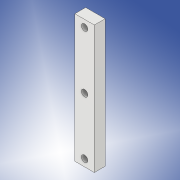
# Autodesk Inventor part: SJ017
Saved by Autodesk Inventor 2017 SP1 (Build 210196100, 196)
## iProperties
Created: 2017-07-22
Part Number: SJ017
Material: ABS Plastic
Document SubType Name: Modeling
Designer: Zach
Density: 1.06 g/cm^3
Appearance: CR White
Author: Zach
Autodesk Inventor part; units mm, degrees
ref_plane "YZ Plane" through (0, 0, 0) normal (1, 0, 0) x (0, 1, 0)
ref_plane "XZ Plane" through (0, 0, 0) normal (0, 1, 0) x (-1, 0, 0)
ref_plane "XY Plane" through (0, 0, 0) normal (0, 0, 1) x (1, 0, 0)
sketch "Sketch1" plane through (0, 0, 0) normal (0, 0, 1) x (1, 0, 0)
  line L0 (0, 0) -> (9, 0)
  line L1 (9, 0) -> (9, 59)
  line L2 (9, 59) -> (0, 59)
  line L3 (0, 59) -> (0, 0)
  circle A0 centre (4.5, 55.75) radius 1.5
  circle A1 centre (4.5, 3.25) radius 1.5
  line L4 (4.5, 55.75) -> (4.5, 3.25) construction
  circle A2 centre (4.5, 29.5) radius 1.5
  point P0 (9, 29.5)
  point P1 (4.5, 59)
  dimension "d0" = 9
  dimension "d1" = 59
  dimension "d2" = 3
  dimension "d3" = 3
  dimension "d4" = 52.5
  dimension "d5" = 3
  constraints: 10 end point, 3 centre point, 3 midpoint, 2 parallel, 2 perpendicular, 1 coincident, 1 horizontal, 1 horizontal alignment, 1 vertical alignment
  measures "d0" distance of L2.end L1.end
  measures "d1" distance of L1.end L0.end
  measures "d2" diameter of A0
  measures "d3" diameter of A1
  measures "d4" distance of L4.start L4.end
  measures "d5" diameter of A2
extrude "Extrusion1" add sketch "Sketch1" along normal blind 5
body "Solid1"
